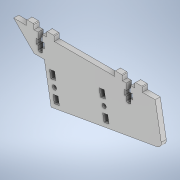
# Autodesk Inventor part: tc_support_front
Saved by Autodesk Inventor 2020 (Build 240168000, 168)
## iProperties
Created: 2019-07-16
Part Number: tc_support_front
Material: Générique
Document SubType Name: Modeling
Designer: Thibault
Density: 1 g/cm^3
Appearance: Par défaut
Author: Thibault
Autodesk Inventor part; units mm, degrees
ref_plane "YZ Plane" through (0, 0, 0) normal (1, 0, 0) x (0, 1, 0)
ref_plane "XZ Plane" through (0, 0, 0) normal (0, 1, 0) x (-1, 0, 0)
ref_plane "XY Plane" through (0, 0, 0) normal (0, 0, 1) x (1, 0, 0)
sketch "Anchor (screw side)" plane through (0, 0, 0) normal (0, 0, 1) x (1, 0, 0)
  circle A0 centre (93.7814, 50.2592) radius 0.85
  line L0 (91.2814, 51.2592) -> (88.2814, 51.2592)
  line L1 (88.2814, 51.2592) -> (88.2814, 49.2592)
  line L2 (88.2814, 49.2592) -> (91.2814, 49.2592)
  line L3 (91.2814, 49.2592) -> (91.2814, 51.2592)
  line L4 (99.2814, 51.2592) -> (96.2814, 51.2592)
  line L5 (96.2814, 51.2592) -> (96.2814, 49.2592)
  line L6 (96.2814, 49.2592) -> (99.2814, 49.2592)
  line L7 (99.2814, 49.2592) -> (99.2814, 51.2592)
  line L8 (91.2814, 51.2592) -> (96.2814, 49.2592) construction
  line L9 (96.2814, 51.2592) -> (91.2814, 49.2592) construction
  line L10 (86.6814, 52.8592) -> (100.8814, 52.8592) construction
  line L11 (100.8814, 52.8592) -> (100.8814, 47.6592) construction
  line L12 (100.8814, 47.6592) -> (86.6814, 47.6592) construction
  line L13 (86.6814, 47.6592) -> (86.6814, 52.8592) construction
  point P0 (103.5798, 50.1132)
  dimension "d27" = 1.7
  dimension "d28" = 3
  dimension "d29" = 2
  dimension "d30" = 3
  dimension "d32" = 5
  dimension "d34" = 1.6
  dimension "d35_1" = 1.6
  dimension "d36_1" = 1.6
  dimension "d37" = 1.6
  measures "d27" diameter of A0
  measures "d28" distance of L2.end L1.end
  measures "d29" distance of L1.end L0.end
  measures "d30" distance of L6.end L5.end
  measures "d32" distance between parallel lines of L5 L3
  measures "d34" distance between parallel lines of L0 L10
  measures "d35_1" distance between parallel lines of L12 L2
  measures "d36_1" distance between parallel lines of L11 L7
  measures "d37" distance between parallel lines of L13 L1
sketch "Anchor (nut side)" plane through (0, 0, 0) normal (0, 0, 1) x (1, 0, 0)
  line L0 (10, 0) -> (8.35, 0)
  line L1 (8.35, 0) -> (8.35, -2.5)
  line L2 (8.35, -2.5) -> (9.15, -2.5)
  line L3 (9.15, -2.5) -> (9.15, -4.5)
  line L4 (5.85, -4.5) -> (5.85, -2.5)
  line L5 (5.85, -2.5) -> (6.65, -2.5)
  line L6 (6.65, -2.5) -> (6.65, 0)
  line L7 (6.65, 0) -> (5, 0)
  line L8 (2, 0) -> (2, 1.75)
  line L9 (2, 0) -> (3, 0) construction
  line L10 (2.25, 2) -> (4.75, 2)
  line L11 (5, 1.75) -> (5, 0)
  line L12 (5, 2) -> (7, 2) construction
  line L13 (10, 0) -> (10, 1.75)
  line L14 (10.25, 2) -> (12.75, 2)
  line L15 (13, 1.75) -> (13, 0)
  line L16 (0, 0) -> (2, 0)
  line L17 (13, 0) -> (15, 0)
  line L18 (5.85, -4.5) -> (6.65, -4.5)
  line L19 (9.15, -4.5) -> (8.35, -4.5)
  line L20 (6.65, -4.5) -> (6.65, -6)
  line L21 (8.35, -4.5) -> (8.35, -6)
  arc A0 (2.25, 2) -> (2, 1.75) centre (2.25, 1.75) ccw
  arc A1 (5, 1.75) -> (4.75, 2) centre (4.75, 1.75) ccw
  arc A2 (10.25, 2) -> (10, 1.75) centre (10.25, 1.75) ccw
  arc A3 (13, 1.75) -> (12.75, 2) centre (12.75, 1.75) ccw
  line L22 (7.15, -6.5) -> (7.85, -6.5)
  arc A4 (6.65, -6) -> (7.15, -6.5) centre (7.15, -6) ccw
  arc A5 (7.85, -6.5) -> (8.35, -6) centre (7.85, -6) ccw
  point P0 (9.1321, -0.6227)
  point P1 (2, 2)
  point P2 (10, 2)
  point P3 (13, 2)
  point P4 (6.65, -6.5)
  point P5 (8.35, -6.5)
  dimension "d3" = 2
  dimension "d5" = 3
  dimension "d7" = 5
  dimension "d8" = 3
  dimension "d10" = 1.65
  dimension "d11" = 2.5
  dimension "d12" = 0.8
  dimension "d13" = 2
  dimension "d14" = 0.8
  dimension "d15" = 1.7
  dimension "d16" = 2.5
  dimension "d18" = 2
  dimension "d19" = 0.8
  dimension "d20" = 0.8
  dimension "d21" = 2
  dimension "d22" = 2
  dimension "d23" = 1.7
  dimension "d24" = 2
  dimension "d25" = 0.25
  dimension "d38" = 2
  dimension "d39_1" = 0.5
  measures "d3" distance of L16.start L8.start
  measures "d5" distance of point (2, 2) L12.start
  measures "d7" distance of L7.end L0.start
  measures "d8" distance of point (10, 2) point (13, 2)
  measures "d10" distance of L0.start L0.end
  measures "d11" distance of L0.end L1.end
  measures "d12" distance of L1.end L2.end
  measures "d13" distance of L2.end L3.end
  measures "d14" distance of L4.end L5.end
  measures "d15" distance of L6.end L0.end
  measures "d16" distance of L5.end L6.end
  measures "d18" distance of L15.end L17.end
  measures "d19" distance of L4.start L18.end
  measures "d20" distance of L3.end L19.end
  measures "d21" distance of L18.end point (6.65, -6.5)
  measures "d22" distance of L19.end point (8.35, -6.5)
  measures "d23" distance of L18.end L19.end
  measures "d24" distance of L4.start L4.end
  measures "d25" radius of A0
  measures "d38" distance between parallel lines of L16 L10
  measures "d39_1" radius of A4
derived "shared_parameters.ipt"
sketch "Esquisse1" plane through (0, 0, 0) normal (0, 0, 1) x (1, 0, 0)
  line L0 (-13.0294, 5.7667) -> (6.9706, 5.7667)
  line L1 (-28.0294, 5.7667) -> (-31.0794, 5.7667)
  line L2 (21.9706, 5.7667) -> (25.0206, 5.7667)
  line L3 (-31.0794, 5.7667) -> (-22.9794, -2.3333)
  line L4 (-31.0794, 5.7667) -> (-19.6242, 5.7667) construction
  line L5 (27.3924, -7.684) -> (25.0206, 5.7667)
  line L6 (-22.9794, -2.3333) -> (-18.9048, -2.3333)
  line L7 (25.77, -10.0009) -> (-16.2465, -17.4096)
  line L8 (-2.0657, -1.8526) -> (7.9343, -1.7975) construction
  line L9 (-16.2465, -17.4096) -> (-18.9048, -2.3333)
  arc A0 (25.77, -10.0009) -> (27.3924, -7.684) centre (25.4227, -8.0313) ccw
  line L10 (-18.0294, 5.7667) -> (-19.6794, 5.7667)
  line L11 (-19.6794, 5.7667) -> (-19.6794, 3.2667)
  line L12 (-19.6794, 3.2667) -> (-18.8794, 3.2667)
  line L13 (-18.8794, 3.2667) -> (-18.8794, 1.2667)
  line L14 (-22.1794, 1.2667) -> (-22.1794, 3.2667)
  line L15 (-22.1794, 3.2667) -> (-21.3794, 3.2667)
  line L16 (-21.3794, 3.2667) -> (-21.3794, 5.7667)
  line L17 (-21.3794, 5.7667) -> (-23.0294, 5.7667)
  line L18 (-26.0294, 5.7667) -> (-26.0294, 7.5167)
  line L19 (-26.0294, 5.7667) -> (-25.0294, 5.7667) construction
  line L20 (-25.7794, 7.7667) -> (-23.2794, 7.7667)
  line L21 (-23.0294, 7.5167) -> (-23.0294, 5.7667)
  line L22 (-23.0294, 7.7667) -> (-21.0294, 7.7667) construction
  line L23 (-18.0294, 5.7667) -> (-18.0294, 7.5167)
  line L24 (-17.7794, 7.7667) -> (-15.2794, 7.7667)
  line L25 (-15.0294, 7.5167) -> (-15.0294, 5.7667)
  line L26 (-28.0294, 5.7667) -> (-26.0294, 5.7667)
  line L27 (-15.0294, 5.7667) -> (-13.0294, 5.7667)
  line L28 (-22.1794, 1.2667) -> (-21.3794, 1.2667)
  line L29 (-18.8794, 1.2667) -> (-19.6794, 1.2667)
  line L30 (-21.3794, 1.2667) -> (-21.3794, -0.2333)
  line L31 (-19.6794, 1.2667) -> (-19.6794, -0.2333)
  arc A1 (-25.7794, 7.7667) -> (-26.0294, 7.5167) centre (-25.7794, 7.5167) ccw
  arc A2 (-23.0294, 7.5167) -> (-23.2794, 7.7667) centre (-23.2794, 7.5167) ccw
  arc A3 (-17.7794, 7.7667) -> (-18.0294, 7.5167) centre (-17.7794, 7.5167) ccw
  arc A4 (-15.0294, 7.5167) -> (-15.2794, 7.7667) centre (-15.2794, 7.5167) ccw
  line L32 (-20.8794, -0.7333) -> (-20.1794, -0.7333)
  arc A5 (-21.3794, -0.2333) -> (-20.8794, -0.7333) centre (-20.8794, -0.2333) ccw
  arc A6 (-20.1794, -0.7333) -> (-19.6794, -0.2333) centre (-20.1794, -0.2333) ccw
  line L33 (16.9706, 5.7667) -> (15.3206, 5.7667)
  line L34 (15.3206, 5.7667) -> (15.3206, 3.2667)
  line L35 (15.3206, 3.2667) -> (16.1206, 3.2667)
  line L36 (16.1206, 3.2667) -> (16.1206, 1.2667)
  line L37 (12.8206, 1.2667) -> (12.8206, 3.2667)
  line L38 (12.8206, 3.2667) -> (13.6206, 3.2667)
  line L39 (13.6206, 3.2667) -> (13.6206, 5.7667)
  line L40 (13.6206, 5.7667) -> (11.9706, 5.7667)
  line L41 (8.9706, 5.7667) -> (8.9706, 7.5167)
  line L42 (8.9706, 5.7667) -> (9.9706, 5.7667) construction
  line L43 (9.2206, 7.7667) -> (11.7206, 7.7667)
  line L44 (11.9706, 7.5167) -> (11.9706, 5.7667)
  line L45 (11.9706, 7.7667) -> (13.9706, 7.7667) construction
  line L46 (16.9706, 5.7667) -> (16.9706, 7.5167)
  line L47 (17.2206, 7.7667) -> (19.7206, 7.7667)
  line L48 (19.9706, 7.5167) -> (19.9706, 5.7667)
  line L49 (6.9706, 5.7667) -> (8.9706, 5.7667)
  line L50 (19.9706, 5.7667) -> (21.9706, 5.7667)
  line L51 (12.8206, 1.2667) -> (13.6206, 1.2667)
  line L52 (16.1206, 1.2667) -> (15.3206, 1.2667)
  line L53 (13.6206, 1.2667) -> (13.6206, -0.2333)
  line L54 (15.3206, 1.2667) -> (15.3206, -0.2333)
  arc A7 (9.2206, 7.7667) -> (8.9706, 7.5167) centre (9.2206, 7.5167) ccw
  arc A8 (11.9706, 7.5167) -> (11.7206, 7.7667) centre (11.7206, 7.5167) ccw
  arc A9 (17.2206, 7.7667) -> (16.9706, 7.5167) centre (17.2206, 7.5167) ccw
  arc A10 (19.9706, 7.5167) -> (19.7206, 7.7667) centre (19.7206, 7.5167) ccw
  line L55 (14.1206, -0.7333) -> (14.8206, -0.7333)
  arc A11 (13.6206, -0.2333) -> (14.1206, -0.7333) centre (14.1206, -0.2333) ccw
  arc A12 (14.8206, -0.7333) -> (15.3206, -0.2333) centre (14.8206, -0.2333) ccw
  circle A13 centre (4.7773, -6.493) radius 0.85
  line L56 (4.2266, -9.1286) -> (4.7475, -12.0831)
  line L57 (4.7475, -12.0831) -> (6.7171, -11.7358)
  line L58 (6.7171, -11.7358) -> (6.1962, -8.7814)
  line L59 (6.1962, -8.7814) -> (4.2266, -9.1286)
  line L60 (2.8374, -1.2502) -> (3.3583, -4.2046)
  line L61 (3.3583, -4.2046) -> (5.3279, -3.8573)
  line L62 (5.3279, -3.8573) -> (4.807, -0.9029)
  line L63 (4.807, -0.9029) -> (2.8374, -1.2502)
  line L64 (4.2266, -9.1286) -> (5.3279, -3.8573) construction
  line L65 (3.3583, -4.2046) -> (6.1962, -8.7814) construction
  line L66 (3.4497, -13.9366) -> (0.9839, 0.0477) construction
  line L67 (0.9839, 0.0477) -> (6.1049, 0.9506) construction
  line L68 (6.1049, 0.9506) -> (8.5707, -13.0336) construction
  line L69 (8.5707, -13.0336) -> (3.4497, -13.9366) construction
  circle A14 centre (-14.9189, -9.9659) radius 0.85
  line L70 (-14.3682, -7.3303) -> (-14.8892, -4.3759)
  line L71 (-14.8892, -4.3759) -> (-16.8588, -4.7232)
  line L72 (-16.8588, -4.7232) -> (-16.3378, -7.6776)
  line L73 (-16.3378, -7.6776) -> (-14.3682, -7.3303)
  line L74 (-12.979, -15.2087) -> (-13.5, -12.2543)
  line L75 (-13.5, -12.2543) -> (-15.4696, -12.6016)
  line L76 (-15.4696, -12.6016) -> (-14.9486, -15.556)
  line L77 (-14.9486, -15.556) -> (-12.979, -15.2087)
  line L78 (-14.3682, -7.3303) -> (-15.4696, -12.6016) construction
  line L79 (-13.5, -12.2543) -> (-16.3378, -7.6776) construction
  line L80 (-13.5913, -2.5223) -> (-11.1255, -16.5066) construction
  line L81 (-11.1255, -16.5066) -> (-16.2465, -17.4096) construction
  line L82 (-16.2465, -17.4096) -> (-18.7123, -3.4253) construction
  line L83 (-18.7123, -3.4253) -> (-13.5913, -2.5223) construction
  point P0 (21.9706, 5.7667)
  point P1 (-13.0294, 5.7667)
  point P2 (27.7396, -9.6536)
  point P3 (22.4992, -2.0098)
  point P4 (4.7773, -6.493)
  point P5 (-14.9189, -9.9659)
  dimension "d2" = 45
  dimension "d26" = 100
  dimension "d33" = 56.1
  dimension "d40" = 1.6
  dimension "d44" = 1.6
  dimension "d45" = 1.6
  dimension "d46" = 2
  dimension "d47" = 20
  constraints: 20 end point, 6 horizontal, 2 equal length, 2 point on circle, 2 point on line, 2 tangent, 1 centre point, 1 parallel, 1 perpendicular, 6 other
  measures "d2" angle of L3 L4
  measures "d26" angle of L5 L2
  measures "d33" distance of L2.end L1.end
  measures "d46" radius of A0
extrude "Extrusion1" add sketch "Esquisse1" along normal blind 2
equation "\"d40\" = safe_distance"
equation "\"d44\" = safe_distance"
equation "\"d45\" = safe_distance"
equation "\"d35\" = sheet_thickness"
equation "\"safe_distance\" = 1.6"
equation "\"sheet_thickness\" = 2"
